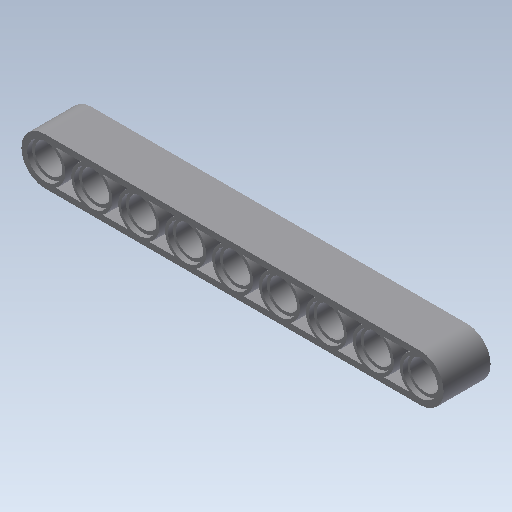
# Autodesk Inventor part: 9M Beam
Saved by Autodesk Inventor 2020 (Build 240168000, 168)
## iProperties
Created: 2014-02-10
Part Number: 9M Beam
Document SubType Name: Modeling
Designer: jleonard
Density: 1 g/cm^3
Material: Generic
Appearance: Default
Author: jleonard
Autodesk Inventor part; units mm, degrees
ref_plane "YZ Plane" through (0, 0, 0) normal (1, 0, 0) x (0, 1, 0)
ref_plane "XZ Plane" through (0, 0, 0) normal (0, 1, 0) x (-1, 0, 0)
ref_plane "XY Plane" through (0, 0, 0) normal (0, 0, 1) x (1, 0, 0)
sketch "Sketch2" plane through (0, 0, 0) normal (0, 0, 1) x (1, 0, 0)
  arc A0 (-32, 4) -> (-32, -4) centre (-32, 0) ccw
  arc A1 (32, -4) -> (32, 4) centre (32, 0) ccw
  line L0 (-32, 4) -> (32, 4)
  line L1 (-32, -4) -> (32, -4)
  line L2 (-50.4, 0) -> (50.4, 0) projected
  line L3 (0, -5.6) -> (0, 5.6) projected
  point P0 (0, 0)
  dimension "d0" = 4
  dimension "d1" = 4
  dimension "d2" = 64
  dimension "d3" = 0
  dimension "d4" = 32
  dimension "d9" = 180
  dimension "d10" = 0
  dimension "d141" = 64
  constraints: 6 point on circle, 4 end point, 2 centre point, 2 point on line, 2 tangent
  measures "d0" radius of A0
  measures "d1" radius of A1
  measures "d2" distance of A1.centre A0.centre
  measures "d3" distance from line of A0.centre L2
  measures "d4" distance from line of A0.centre L3
  measures "d9" angle of L0 L2
  measures "d10" distance from line of L2 A1.centre
  measures "d141" distance of L1.start L1.end
extrude "Extrusion1" add sketch "Sketch2" along normal blind 8
sketch "Sketch15" plane through (0, 0, 8) normal (0, 0, 1) x (1, 0, 0)
  arc A0 (-32, 4) -> (-32, -4) centre (-32, 0) ccw projected
  circle A1 centre (-32, 0) radius 2.5
  line L0 (-50.4, 0) -> (50.4, 0) projected
  circle A2 centre (-24, 0) radius 2.5
  circle A3 centre (-16, 0) radius 2.5
  circle A4 centre (-8, 0) radius 2.5
  circle A5 centre (0, 0) radius 2.5
  circle A6 centre (8, 0) radius 2.5
  circle A7 centre (16, 0) radius 2.5
  circle A8 centre (24, 0) radius 2.5
  circle A9 centre (32, 0) radius 2.5
  dimension "d142" = 5
  dimension "d148" = 8
  constraints: 9 centre point, 1 coincident, 1 horizontal, 16 other
  measures "d142" diameter of A1
  measures "d148" distance of A1.centre A2.centre
extrude "Extrusion14" cut sketch "Sketch15" against normal through all
sketch "Sketch16" plane through (0, 0, 8) normal (0, 0, 1) x (1, 0, 0)
  circle A0 centre (32, 0) radius 2.5 projected
  circle A1 centre (24, 0) radius 2.5 projected
  circle A2 centre (16, 0) radius 2.5 projected
  circle A3 centre (8, 0) radius 2.5 projected
  circle A4 centre (0, 0) radius 2.5 projected
  circle A5 centre (-8, 0) radius 2.5 projected
  circle A6 centre (-16, 0) radius 2.5 projected
  circle A7 centre (-24, 0) radius 2.5 projected
  circle A8 centre (-32, 0) radius 2.5 projected
  arc A9 (-32, 4) -> (-32, -4) centre (-32, 0) ccw projected
  circle A10 centre (-32, 0) radius 3
  line L0 (-50.4, 0) -> (50.4, 0) projected
  circle A11 centre (-24, 0) radius 3
  circle A12 centre (-16, 0) radius 3
  circle A13 centre (-8, 0) radius 3
  circle A14 centre (0, 0) radius 3
  circle A15 centre (8, 0) radius 3
  circle A16 centre (16, 0) radius 3
  circle A17 centre (24, 0) radius 3
  circle A18 centre (32, 0) radius 3
  dimension "d152" = 6
  dimension "d158" = 8
  constraints: 9 centre point, 1 coincident, 1 horizontal, 16 other
  measures "d152" diameter of A10
  measures "d158" distance of A10.centre A11.centre
extrude "Extrusion15" cut sketch "Sketch16" against normal blind 0.8 contours L0 A18 A0 | A0 L0 A18 | A10 L0 A8 | L0 A8 A10 | A11 L0 A7 | L0 A7 A11 | A12 L0 A6 | L0 A6 A12 | A13 L0 A5 | L0 A5 A13 | A14 L0 A4 | L0 A4 A14 | A15 L0 A3 | L0 A3 A15 | A16 L0 A2 | L0 A2 A16 | A17 L0 A1 | L0 A1 A17
sketch "Sketch17" plane through (0, 0, 0) normal (0, 0, -1) x (-1, 0, 0)
  circle A0 centre (-32, 0) radius 2.5 projected
  circle A1 centre (-24, 0) radius 2.5 projected
  circle A2 centre (-16, 0) radius 2.5 projected
  circle A3 centre (-8, 0) radius 2.5 projected
  circle A4 centre (0, 0) radius 2.5 projected
  circle A5 centre (8, 0) radius 2.5 projected
  circle A6 centre (16, 0) radius 2.5 projected
  circle A7 centre (24, 0) radius 2.5 projected
  circle A8 centre (32, 0) radius 2.5 projected
  arc A9 (-32, 4) -> (-32, -4) centre (-32, 0) ccw projected
  circle A10 centre (-32, 0) radius 3
  line L0 (50.4, 0) -> (-50.4, 0) projected
  circle A11 centre (-24, 0) radius 3
  circle A12 centre (-16, 0) radius 3
  circle A13 centre (-8, 0) radius 3
  circle A14 centre (0, 0) radius 3
  circle A15 centre (8, 0) radius 3
  circle A16 centre (16, 0) radius 3
  circle A17 centre (24, 0) radius 3
  circle A18 centre (32, 0) radius 3
  dimension "d162" = 6
  dimension "d168" = 8
  constraints: 9 centre point, 1 coincident, 1 horizontal, 16 other
  measures "d162" diameter of A10
  measures "d168" distance of A10.centre A11.centre
extrude "Extrusion16" cut sketch "Sketch17" against normal blind 0.8 contours L0 A10 A0 | A0 L0 A10 | A18 L0 A8 | L0 A8 A18 | A17 L0 A7 | L0 A7 A17 | A16 L0 A6 | L0 A6 A16 | A15 L0 A5 | L0 A5 A15 | A14 L0 A4 | L0 A4 A14 | A13 L0 A3 | L0 A3 A13 | A12 L0 A2 | L0 A2 A12 | A11 L0 A1 | L0 A1 A11
sketch "Sketch18" plane through (0, 0, 8) normal (0, 0, 1) x (1, 0, 0)
  circle A0 centre (-32, 0) radius 3 projected
  circle A1 centre (-24, 0) radius 3 projected
  arc A2 (-32, 4) -> (-32, -4) centre (-32, 0) ccw projected
  line L0 (-32, 4) -> (32, 4) projected
  arc A3 (-30.1972, -3) -> (-30.1972, 3) centre (-32, 0) ccw
  arc A4 (-25.8028, 3) -> (-25.8028, -3) centre (-24, 0) ccw
  line L1 (-30.1972, 3) -> (-25.8028, 3)
  line L2 (-25.8028, -3) -> (-30.1972, -3)
  line L3 (-50.4, 0) -> (50.4, 0) projected
  arc A5 (-22.1972, -3) -> (-22.1972, 3) centre (-24, 0) ccw
  arc A6 (-17.8028, 3) -> (-17.8028, -3) centre (-16, 0) ccw
  line L4 (-22.1972, 3) -> (-17.8028, 3)
  line L5 (-17.8028, -3) -> (-22.1972, -3)
  arc A7 (-14.1972, -3) -> (-14.1972, 3) centre (-16, 0) ccw
  arc A8 (-9.8028, 3) -> (-9.8028, -3) centre (-8, 0) ccw
  line L6 (-14.1972, 3) -> (-9.8028, 3)
  line L7 (-9.8028, -3) -> (-14.1972, -3)
  arc A9 (-6.1972, -3) -> (-6.1972, 3) centre (-8, 0) ccw
  arc A10 (-1.8028, 3) -> (-1.8028, -3) centre (0, 0) ccw
  line L8 (-6.1972, 3) -> (-1.8028, 3)
  line L9 (-1.8028, -3) -> (-6.1972, -3)
  arc A11 (1.8028, -3) -> (1.8028, 3) centre (0, 0) ccw
  arc A12 (6.1972, 3) -> (6.1972, -3) centre (8, 0) ccw
  line L10 (1.8028, 3) -> (6.1972, 3)
  line L11 (6.1972, -3) -> (1.8028, -3)
  arc A13 (9.8028, -3) -> (9.8028, 3) centre (8, 0) ccw
  arc A14 (14.1972, 3) -> (14.1972, -3) centre (16, 0) ccw
  line L12 (9.8028, 3) -> (14.1972, 3)
  line L13 (14.1972, -3) -> (9.8028, -3)
  arc A15 (17.8028, -3) -> (17.8028, 3) centre (16, 0) ccw
  arc A16 (22.1972, 3) -> (22.1972, -3) centre (24, 0) ccw
  line L14 (17.8028, 3) -> (22.1972, 3)
  line L15 (22.1972, -3) -> (17.8028, -3)
  arc A17 (25.8028, -3) -> (25.8028, 3) centre (24, 0) ccw
  arc A18 (30.1972, 3) -> (30.1972, -3) centre (32, 0) ccw
  line L16 (25.8028, 3) -> (30.1972, 3)
  line L17 (30.1972, -3) -> (25.8028, -3)
  dimension "d172" = 7
  dimension "d173" = 7
  dimension "d179" = 8
  constraints: 32 end point, 32 point on circle, 16 centre point, 3 tangent, 2 coincident, 1 horizontal, 1 parallel, 70 other
  measures "d172" diameter of A3
  measures "d173" diameter of A4
  measures "d179" distance of L1.start L4.start
extrude "Extrusion17" cut sketch "Sketch18" against normal through all contours A17 L16 A18 L3 | L3 A18 L17 A17 | A15 L14 A16 L3 | L3 A16 L15 A15 | A13 L12 A14 L3 | L3 A14 L13 A13 | A11 L10 A12 L3 | L3 A12 L11 A11 | A9 L8 A10 L3 | L3 A10 L9 A9 | A7 L6 A8 L3 | L3 A8 L7 A7 | A5 L4 A6 L3 | L3 A6 L5 A5 | A3 L1 A4 L3 | L3 A4 L2 A3
body "Solid1"
